Autodesk Fusion 360 part; units mm, degrees
(part 4 of 5)
  spline S150 degree 3 poles (259.5446, 19.7544) (259.234, 19.2928) (259.0786, 18.738) (259.0786, 18.09) knots 0 0 0 0 1 1 1 1
  spline S151 degree 3 poles (259.0786, 18.09) (259.0786, 17.4509) (259.2296, 16.9716) (259.5313, 16.652) knots 0 0 0 0 1 1 1 1
  spline S152 degree 3 poles (259.5313, 16.652) (259.8421, 16.3413) (260.2237, 16.186) (260.6763, 16.186) knots 0 0 0 0 1 1 1 1
  spline S153 degree 3 poles (260.6763, 16.186) (261.3421, 16.186) (261.9812, 16.4168) (262.5937, 16.8784) knots 0 0 0 0 1 1 1 1
  spline S154 degree 3 poles (262.5937, 16.8784) (263.2062, 17.34) (263.7034, 17.9435) (264.0849, 18.6892) knots 0 0 0 0 1 1 1 1
  spline S155 degree 3 poles (264.0849, 18.6892) (264.2803, 18.5028) (264.4577, 18.272) (264.6175, 17.9968) knots 0 0 0 0 1 1 1 1
  spline S156 degree 3 poles (264.6175, 17.9968) (264.3246, 17.3311) (263.8053, 16.6786) (263.0597, 16.0395) knots 0 0 0 0 1 1 1 1
  spline S157 degree 3 poles (263.0597, 16.0395) (262.6869, 15.7289) (262.2431, 15.4759) (261.7282, 15.2806) knots 0 0 0 0 1 1 1 1
  spline S158 degree 3 poles (261.7282, 15.2806) (261.2223, 15.0853) (260.6986, 14.9877) (260.1571, 14.9877) knots 0 0 0 0 1 1 1 1
  spline S159 degree 3 poles (260.1571, 14.9877) (259.2694, 14.9877) (258.5682, 15.2584) (258.0533, 15.7999) knots 0 0 0 0 1 1 1 1
  spline S160 degree 3 poles (258.0533, 15.7999) (257.5031, 16.3857) (257.2278, 17.1358) (257.2278, 18.0501) knots 0 0 0 0 1 1 1 1
  spline S161 degree 3 poles (257.2278, 18.0501) (257.2278, 18.9644) (257.5696, 19.7632) (258.2531, 20.4467) knots 0 0 0 0 1 1 1 1
  spline S162 degree 3 poles (258.2531, 20.4467) (258.9454, 21.1302) (259.7709, 21.472) (260.7296, 21.472) knots 0 0 0 0 1 1 1 1
  spline S163 degree 3 poles (260.7296, 21.472) (261.4132, 21.472) (261.9679, 21.3211) (262.394, 21.0193) knots 0 0 0 0 1 1 1 1
  spline S164 degree 3 poles (262.394, 21.0193) (262.82, 20.7263) (263.0376, 20.3269) (263.0464, 19.8209) knots 0 0 0 0 1 1 1 1
  spline S165 degree 3 poles (263.0464, 19.8209) (263.0464, 19.1374) (262.7713, 18.5827) (262.2209, 18.1566) knots 0 0 0 0 1 1 1 1
  spline S166 degree 3 poles (262.2209, 18.1566) (261.6795, 17.7305) (260.9339, 17.4332) (259.984, 17.2645) knots 0 0 0 0 1 1 1 1
  line L27 (259.984, 17.2645) -> (259.7976, 18.0501)
  spline S167 degree 3 poles (264.5353, 24.8672) (264.7394, 25.0803) (264.988, 25.1868) (265.281, 25.1868) knots 0 0 0 0 1 1 1 1
  spline S168 degree 3 poles (265.281, 25.1868) (265.5739, 25.1868) (265.8223, 25.0803) (266.0266, 24.8672) knots 0 0 0 0 1 1 1 1
  spline S169 degree 3 poles (266.0266, 24.8672) (266.2396, 24.6631) (266.3461, 24.4145) (266.3461, 24.1216) knots 0 0 0 0 1 1 1 1
  spline S170 degree 3 poles (266.3461, 24.1216) (266.3461, 23.8287) (266.2396, 23.5801) (266.0266, 23.376) knots 0 0 0 0 1 1 1 1
  spline S171 degree 3 poles (266.0266, 23.376) (265.8223, 23.1718) (265.5739, 23.0697) (265.281, 23.0697) knots 0 0 0 0 1 1 1 1
  spline S172 degree 3 poles (265.281, 23.0697) (264.988, 23.0697) (264.7394, 23.1718) (264.5353, 23.376) knots 0 0 0 0 1 1 1 1
  spline S173 degree 3 poles (264.5353, 23.376) (264.3311, 23.5801) (264.2291, 23.8287) (264.2291, 24.1216) knots 0 0 0 0 1 1 1 1
  spline S174 degree 3 poles (264.2291, 24.1216) (264.2291, 24.4145) (264.3311, 24.6631) (264.5353, 24.8672) knots 0 0 0 0 1 1 1 1
  spline S175 degree 3 poles (263.9894, 20.966) (264.0781, 21.1258) (264.2468, 21.2456) (264.4954, 21.3255) knots 0 0 0 0 1 1 1 1
  spline S176 degree 3 poles (264.4954, 21.3255) (264.7438, 21.4143) (264.988, 21.4586) (265.2277, 21.4586) knots 0 0 0 0 1 1 1 1
  spline S177 degree 3 poles (265.2277, 21.4586) (265.4761, 21.4586) (265.6937, 21.4276) (265.8801, 21.3654) knots 0 0 0 0 1 1 1 1
  spline S178 degree 3 poles (265.8801, 21.3654) (265.5339, 18.6936) (265.3609, 17.3444) (265.3609, 17.3178) knots 0 0 0 0 1 1 1 1
  spline S179 degree 3 poles (265.3609, 17.3178) (265.3163, 17.1402) (265.2943, 16.9893) (265.2943, 16.8651) knots 0 0 0 0 1 1 1 1
  spline S180 degree 3 poles (265.2943, 16.8651) (265.2943, 16.7497) (265.303, 16.6476) (265.3209, 16.5588) knots 0 0 0 0 1 1 1 1
  spline S181 degree 3 poles (265.3209, 16.5588) (265.3563, 16.328) (265.5161, 16.2126) (265.8002, 16.2126) knots 0 0 0 0 1 1 1 1
  spline S182 degree 3 poles (265.8002, 16.2126) (266.0932, 16.2126) (266.3595, 16.399) (266.5991, 16.7719) knots 0 0 0 0 1 1 1 1
  spline S183 degree 3 poles (266.5991, 16.7719) (266.8475, 17.1535) (267.0339, 17.584) (267.1583, 18.0634) knots 0 0 0 0 1 1 1 1
  spline S184 degree 3 poles (267.1583, 18.0634) (267.2204, 18.0279) (267.3181, 17.9214) (267.4513, 17.7438) knots 0 0 0 0 1 1 1 1
  spline S185 degree 3 poles (267.4513, 17.7438) (267.5844, 17.5663) (267.6643, 17.4332) (267.6909, 17.3444) knots 0 0 0 0 1 1 1 1
  spline S186 degree 3 poles (267.6909, 17.3444) (267.5133, 16.6343) (267.2116, 16.0617) (266.7855, 15.6268) knots 0 0 0 0 1 1 1 1
  spline S187 degree 3 poles (266.7855, 15.6268) (266.3595, 15.1918) (265.8489, 14.9744) (265.2543, 14.9744) knots 0 0 0 0 1 1 1 1
  spline S188 degree 3 poles (265.2543, 14.9744) (264.6596, 14.9744) (264.2158, 15.1208) (263.9229, 15.4137) knots 0 0 0 0 1 1 1 1
  spline S189 degree 3 poles (263.9229, 15.4137) (263.6387, 15.7067) (263.4968, 16.0839) (263.4968, 16.5455) knots 0 0 0 0 1 1 1 1
  spline S190 degree 3 poles (263.4968, 16.5455) (263.4968, 16.6431) (263.5012, 16.7452) (263.5101, 16.8517) knots 0 0 0 0 1 1 1 1
  line L28 (263.5101, 16.8517) -> (263.9894, 20.966)
  line L29 (270.3997, 16.5588) -> (270.7193, 19.528)
  spline S191 degree 3 poles (270.7193, 19.528) (270.7193, 19.7677) (270.6571, 19.9674) (270.5329, 20.1272) knots 0 0 0 0 1 1 1 1
  spline S192 degree 3 poles (270.5329, 20.1272) (270.4085, 20.2869) (270.2, 20.3668) (269.9071, 20.3668) knots 0 0 0 0 1 1 1 1
  spline S193 degree 3 poles (269.9071, 20.3668) (269.6229, 20.3668) (269.3789, 20.2381) (269.1748, 19.9807) knots 0 0 0 0 1 1 1 1
  spline S194 degree 3 poles (269.1748, 19.9807) (268.9794, 19.7322) (268.8552, 19.4171) (268.802, 19.0354) knots 0 0 0 0 1 1 1 1
  spline S195 degree 3 poles (268.802, 19.0354) (268.4824, 16.6032) (268.3137, 15.2806) (268.296, 15.0676) knots 0 0 0 0 1 1 1 1
  line L30 (268.296, 15.0676) -> (266.4985, 15.0676)
  line L31 (266.4985, 15.0676) -> (267.2308, 21.3388)
  spline S196 degree 3 poles (267.2308, 21.3388) (267.6036, 21.4365) (267.8876, 21.4853) (268.083, 21.4853) knots 0 0 0 0 1 1 1 1
  spline S197 degree 3 poles (268.083, 21.4853) (268.6776, 21.4853) (268.9884, 21.2678) (269.015, 20.8328) knots 0 0 0 0 1 1 1 1
  spline S198 degree 3 poles (269.015, 20.8328) (269.4498, 21.2589) (269.9691, 21.472) (270.5728, 21.472) knots 0 0 0 0 1 1 1 1
  spline S199 degree 3 poles (270.5728, 21.472) (271.1853, 21.472) (271.6646, 21.3211) (272.0108, 21.0193) knots 0 0 0 0 1 1 1 1
  spline S200 degree 3 poles (272.0108, 21.0193) (272.357, 20.7175) (272.5301, 20.3358) (272.5301, 19.8742) knots 0 0 0 0 1 1 1 1
  spline S201 degree 3 poles (272.5301, 19.8742) (272.5301, 19.7499) (272.5035, 19.5147) (272.4502, 19.1685) knots 0 0 0 0 1 1 1 1
  spline S202 degree 3 poles (272.4502, 19.1685) (272.2459, 17.8193) (272.144, 17.0337) (272.144, 16.8118) knots 0 0 0 0 1 1 1 1
  spline S203 degree 3 poles (272.144, 16.8118) (272.144, 16.4035) (272.2815, 16.1993) (272.5567, 16.1993) knots 0 0 0 0 1 1 1 1
  spline S204 degree 3 poles (272.5567, 16.1993) (273.1602, 16.1993) (273.6173, 16.8296) (273.9281, 18.09) knots 0 0 0 0 1 1 1 1
  spline S205 degree 3 poles (273.9281, 18.09) (274.2298, 17.7705) (274.4118, 17.5175) (274.474, 17.3311) knots 0 0 0 0 1 1 1 1
  spline S206 degree 3 poles (274.474, 17.3311) (274.0035, 15.7688) (273.1869, 14.9877) (272.0241, 14.9877) knots 0 0 0 0 1 1 1 1
  spline S207 degree 3 poles (272.0241, 14.9877) (271.4737, 14.9877) (271.0655, 15.1563) (270.7992, 15.4936) knots 0 0 0 0 1 1 1 1
  spline S208 degree 3 poles (270.7992, 15.4936) (270.5329, 15.831) (270.3997, 16.186) (270.3997, 16.5588) knots 0 0 0 0 1 1 1 1
  spline S209 degree 3 poles (275.986, 18.0501) (276.5363, 18.1655) (276.9447, 18.3874) (277.211, 18.7158) knots 0 0 0 0 1 1 1 1
  spline S210 degree 3 poles (277.211, 18.7158) (277.486, 19.0442) (277.6237, 19.3594) (277.6237, 19.6611) knots 0 0 0 0 1 1 1 1
  spline S211 degree 3 poles (277.6237, 19.6611) (277.6237, 19.9718) (277.5393, 20.1804) (277.3708, 20.2869) knots 0 0 0 0 1 1 1 1
  spline S212 degree 3 poles (277.3708, 20.2869) (277.211, 20.4023) (277.0333, 20.46) (276.8382, 20.46) knots 0 0 0 0 1 1 1 1
  spline S213 degree 3 poles (276.8382, 20.46) (276.4208, 20.46) (276.0526, 20.2248) (275.733, 19.7544) knots 0 0 0 0 1 1 1 1
  spline S214 degree 3 poles (275.733, 19.7544) (275.4222, 19.2928) (275.267, 18.738) (275.267, 18.09) knots 0 0 0 0 1 1 1 1
  spline S215 degree 3 poles (275.267, 18.09) (275.267, 17.4509) (275.4179, 16.9716) (275.7197, 16.652) knots 0 0 0 0 1 1 1 1
  spline S216 degree 3 poles (275.7197, 16.652) (276.0303, 16.3413) (276.4121, 16.186) (276.8648, 16.186) knots 0 0 0 0 1 1 1 1
  spline S217 degree 3 poles (276.8648, 16.186) (277.5305, 16.186) (278.1696, 16.4168) (278.7821, 16.8784) knots 0 0 0 0 1 1 1 1
  spline S218 degree 3 poles (278.7821, 16.8784) (279.3946, 17.34) (279.8916, 17.9435) (280.2734, 18.6892) knots 0 0 0 0 1 1 1 1
  spline S219 degree 3 poles (280.2734, 18.6892) (280.4685, 18.5028) (280.6462, 18.272) (280.806, 17.9968) knots 0 0 0 0 1 1 1 1
  spline S220 degree 3 poles (280.806, 17.9968) (280.513, 17.3311) (279.9938, 16.6786) (279.2481, 16.0395) knots 0 0 0 0 1 1 1 1
  spline S221 degree 3 poles (279.2481, 16.0395) (278.8753, 15.7289) (278.4314, 15.4759) (277.9167, 15.2806) knots 0 0 0 0 1 1 1 1
  spline S222 degree 3 poles (277.9167, 15.2806) (277.4107, 15.0853) (276.8869, 14.9877) (276.3455, 14.9877) knots 0 0 0 0 1 1 1 1
  spline S223 degree 3 poles (276.3455, 14.9877) (275.4578, 14.9877) (274.7565, 15.2584) (274.2418, 15.7999) knots 0 0 0 0 1 1 1 1
  spline S224 degree 3 poles (274.2418, 15.7999) (273.6913, 16.3857) (273.4163, 17.1358) (273.4163, 18.0501) knots 0 0 0 0 1 1 1 1
  spline S225 degree 3 poles (273.4163, 18.0501) (273.4163, 18.9644) (273.7579, 19.7632) (274.4415, 20.4467) knots 0 0 0 0 1 1 1 1
  spline S226 degree 3 poles (274.4415, 20.4467) (275.1339, 21.1302) (275.9594, 21.472) (276.9181, 21.472) knots 0 0 0 0 1 1 1 1
  spline S227 degree 3 poles (276.9181, 21.472) (277.6015, 21.472) (278.1563, 21.3211) (278.5824, 21.0193) knots 0 0 0 0 1 1 1 1
  spline S228 degree 3 poles (278.5824, 21.0193) (279.0085, 20.7263) (279.2259, 20.3269) (279.2348, 19.8209) knots 0 0 0 0 1 1 1 1
  spline S229 degree 3 poles (279.2348, 19.8209) (279.2348, 19.1374) (278.9596, 18.5827) (278.4093, 18.1566) knots 0 0 0 0 1 1 1 1
  spline S230 degree 3 poles (278.4093, 18.1566) (277.8678, 17.7305) (277.1221, 17.4332) (276.1724, 17.2645) knots 0 0 0 0 1 1 1 1
  line L32 (276.1724, 17.2645) -> (275.986, 18.0501)
  line L33 (231.6876, 10.7897) -> (231.6743, 10.6167)
  spline S231 degree 3 poles (231.6743, 10.6167) (231.337, 8.0247) (231.1151, 6.4269) (231.0085, 5.8233) knots 0 0 0 0 1 1 1 1
  spline S232 degree 3 poles (231.0085, 5.8233) (230.831, 4.8291) (230.7423, 4.0702) (230.7423, 3.5465) knots 0 0 0 0 1 1 1 1
  spline S233 degree 3 poles (230.7423, 3.5465) (230.7423, 3.0316) (230.9642, 2.7743) (231.408, 2.7743) knots 0 0 0 0 1 1 1 1
  spline S234 degree 3 poles (231.408, 2.7743) (231.7808, 2.7743) (232.1137, 3.0406) (232.4066, 3.5731) knots 0 0 0 0 1 1 1 1
  spline S235 degree 3 poles (232.4066, 3.5731) (232.6995, 4.1147) (232.9214, 4.7848) (233.0723, 5.5837) knots 0 0 0 0 1 1 1 1
  spline S236 degree 3 poles (233.0723, 5.5837) (233.383, 7.2525) (233.5383, 8.6949) (233.5383, 9.911) knots 0 0 0 0 1 1 1 1
  spline S237 degree 3 poles (233.5383, 9.911) (233.5383, 10.4791) (233.4895, 10.9717) (233.3919, 11.3889) knots 0 0 0 0 1 1 1 1
  spline S238 degree 3 poles (233.3919, 11.3889) (233.747, 11.6019) (234.173, 11.7085) (234.6701, 11.7085) knots 0 0 0 0 1 1 1 1
  spline S239 degree 3 poles (234.6701, 11.7085) (235.1672, 11.7085) (235.4157, 11.4155) (235.4157, 10.8297) knots 0 0 0 0 1 1 1 1
  spline S240 degree 3 poles (235.4157, 10.8297) (235.4157, 9.9154) (235.2737, 8.5262) (234.9897, 6.6622) knots 0 0 0 0 1 1 1 1
  spline S241 degree 3 poles (234.9897, 6.6622) (234.7589, 5.1087) (234.4393, 3.9682) (234.031, 3.2403) knots 0 0 0 0 1 1 1 1
  spline S242 degree 3 poles (234.031, 3.2403) (233.8446, 2.9297) (233.6316, 2.6322) (233.3919, 2.3482) knots 0 0 0 0 1 1 1 1
  spline S243 degree 3 poles (233.3919, 2.3482) (232.8948, 1.7713) (232.198, 1.4827) (231.3015, 1.4827) knots 0 0 0 0 1 1 1 1
  spline S244 degree 3 poles (231.3015, 1.4827) (230.4138, 1.4827) (229.7792, 1.8645) (229.3975, 2.6278) knots 0 0 0 0 1 1 1 1
  spline S245 degree 3 poles (229.3975, 2.6278) (228.9093, 1.8645) (228.1681, 1.4827) (227.1739, 1.4827) knots 0 0 0 0 1 1 1 1
  spline S246 degree 3 poles (227.1739, 1.4827) (226.5348, 1.4827) (226.0377, 1.6648) (225.6827, 2.0286) knots 0 0 0 0 1 1 1 1
  spline S247 degree 3 poles (225.6827, 2.0286) (225.3365, 2.4014) (225.1634, 2.8941) (225.1634, 3.5066) knots 0 0 0 0 1 1 1 1
  spline S248 degree 3 poles (225.1634, 3.5066) (225.1634, 3.5865) (225.1723, 3.7063) (225.19, 3.8661) knots 0 0 0 0 1 1 1 1
  line L34 (225.19, 3.8661) -> (225.6827, 7.6208)
  spline S249 degree 3 poles (225.6827, 7.6208) (224.7329, 8.3043) (224.258, 9.0721) (224.258, 9.9243) knots 0 0 0 0 1 1 1 1
  spline S250 degree 3 poles (224.258, 9.9243) (224.258, 10.4658) (224.4444, 10.8963) (224.8172, 11.2158) knots 0 0 0 0 1 1 1 1
  spline S251 degree 3 poles (224.8172, 11.2158) (225.19, 11.5354) (225.6427, 11.6952) (226.1753, 11.6952) knots 0 0 0 0 1 1 1 1
  spline S252 degree 3 poles (226.1753, 11.6952) (227.3381, 11.6952) (227.9195, 11.1182) (227.9195, 9.9642) knots 0 0 0 0 1 1 1 1
  spline S253 degree 3 poles (227.9195, 9.9642) (227.9195, 9.9465) (227.9151, 9.9243) (227.9062, 9.8977) knots 0 0 0 0 1 1 1 1
  spline S254 degree 3 poles (227.9062, 9.8977) (227.9062, 9.871) (227.9018, 9.8267) (227.8929, 9.7645) knots 0 0 0 0 1 1 1 1
  spline S255 degree 3 poles (227.8929, 9.7645) (227.8929, 9.7113) (227.884, 9.6447) (227.8663, 9.5648) knots 0 0 0 0 1 1 1 1
  spline S256 degree 3 poles (227.8663, 9.5648) (227.8574, 9.4938) (227.8396, 9.3828) (227.813, 9.2319) knots 0 0 0 0 1 1 1 1
  spline S257 degree 3 poles (227.813, 9.2319) (227.7953, 9.081) (227.7731, 8.9124) (227.7464, 8.726) knots 0 0 0 0 1 1 1 1
  spline S258 degree 3 poles (227.7464, 8.726) (227.7198, 8.5484) (227.6843, 8.3088) (227.6399, 8.007) knots 0 0 0 0 1 1 1 1
  spline S259 degree 3 poles (227.6399, 8.007) (227.5955, 7.7052) (227.5467, 7.3767) (227.4935, 7.0217) knots 0 0 0 0 1 1 1 1
  spline S260 degree 3 poles (227.4935, 7.0217) (227.4491, 6.6755) (227.3914, 6.2494) (227.3204, 5.7434) knots 0 0 0 0 1 1 1 1
  spline S261 degree 3 poles (227.3204, 5.7434) (227.2494, 5.2375) (227.1872, 4.807) (227.134, 4.4519) knots 0 0 0 0 1 1 1 1
  spline S262 degree 3 poles (227.134, 4.4519) (227.0807, 4.0968) (227.0541, 3.8394) (227.0541, 3.6797) knots 0 0 0 0 1 1 1 1
  spline S263 degree 3 poles (227.0541, 3.6797) (227.0541, 3.0849) (227.2849, 2.7876) (227.7464, 2.7876) knots 0 0 0 0 1 1 1 1
  spline S264 degree 3 poles (227.7464, 2.7876) (228.3855, 2.7876) (228.7806, 3.369) (228.9314, 4.5318) knots 0 0 0 0 1 1 1 1
  line L35 (228.9314, 4.5318) -> (229.7836, 11.2558)
  spline S265 degree 3 poles (229.7836, 11.2558) (230.0765, 11.3889) (230.4271, 11.4555) (230.8355, 11.4555) knots 0 0 0 0 1 1 1 1
  spline S266 degree 3 poles (230.8355, 11.4555) (231.4036, 11.4555) (231.6876, 11.2336) (231.6876, 10.7897) knots 0 0 0 0 1 1 1 1
  spline S267 degree 3 poles (225.656, 10.63) (225.4874, 10.63) (225.3631, 10.5678) (225.2832, 10.4436) knots 0 0 0 0 1 1 1 1
  spline S268 degree 3 poles (225.2832, 10.4436) (225.2033, 10.3193) (225.1634, 10.1773) (225.1634, 10.0175) knots 0 0 0 0 1 1 1 1
  spline S269 degree 3 poles (225.1634, 10.0175) (225.1634, 9.6181) (225.3853, 9.2053) (225.8291, 8.7792) knots 0 0 0 0 1 1 1 1
  line L36 (225.8291, 8.7792) -> (225.8957, 9.3118)
  spline S270 degree 3 poles (225.8957, 9.3118) (225.9312, 9.6047) (225.9489, 9.8977) (225.9489, 10.1906) knots 0 0 0 0 1 1 1 1
  spline S271 degree 3 poles (225.9489, 10.1906) (225.9578, 10.4835) (225.8602, 10.63) (225.656, 10.63) knots 0 0 0 0 1 1 1 1
  spline S272 degree 3 poles (238.1872, 4.5451) (238.7375, 4.6606) (239.1458, 4.8824) (239.4121, 5.2109) knots 0 0 0 0 1 1 1 1
  spline S273 degree 3 poles (239.4121, 5.2109) (239.6874, 5.5393) (239.8249, 5.8543) (239.8249, 6.1562) knots 0 0 0 0 1 1 1 1
  spline S274 degree 3 poles (239.8249, 6.1562) (239.8249, 6.4669) (239.7406, 6.6755) (239.5719, 6.782) knots 0 0 0 0 1 1 1 1
  spline S275 degree 3 poles (239.5719, 6.782) (239.4121, 6.8974) (239.2347, 6.9551) (239.0393, 6.9551) knots 0 0 0 0 1 1 1 1
  spline S276 degree 3 poles (239.0393, 6.9551) (238.6221, 6.9551) (238.2537, 6.7199) (237.9342, 6.2494) knots 0 0 0 0 1 1 1 1
  spline S277 degree 3 poles (237.9342, 6.2494) (237.6235, 5.7878) (237.4682, 5.2331) (237.4682, 4.5851) knots 0 0 0 0 1 1 1 1
  spline S278 degree 3 poles (237.4682, 4.5851) (237.4682, 3.946) (237.6191, 3.4666) (237.9209, 3.1471) knots 0 0 0 0 1 1 1 1
  spline S279 degree 3 poles (237.9209, 3.1471) (238.2315, 2.8365) (238.6132, 2.6811) (239.066, 2.6811) knots 0 0 0 0 1 1 1 1
  spline S280 degree 3 poles (239.066, 2.6811) (239.7317, 2.6811) (240.3708, 2.9118) (240.9833, 3.3734) knots 0 0 0 0 1 1 1 1
  spline S281 degree 3 poles (240.9833, 3.3734) (241.5958, 3.8351) (242.0928, 4.4386) (242.4745, 5.1842) knots 0 0 0 0 1 1 1 1
  spline S282 degree 3 poles (242.4745, 5.1842) (242.6699, 4.9978) (242.8473, 4.7671) (243.0071, 4.4919) knots 0 0 0 0 1 1 1 1
  spline S283 degree 3 poles (243.0071, 4.4919) (242.7142, 3.8261) (242.1949, 3.1737) (241.4493, 2.5346) knots 0 0 0 0 1 1 1 1
  spline S284 degree 3 poles (241.4493, 2.5346) (241.0765, 2.224) (240.6327, 1.971) (240.1178, 1.7757) knots 0 0 0 0 1 1 1 1
  spline S285 degree 3 poles (240.1178, 1.7757) (239.6119, 1.5803) (239.0882, 1.4827) (238.5467, 1.4827) knots 0 0 0 0 1 1 1 1
  spline S286 degree 3 poles (238.5467, 1.4827) (237.659, 1.4827) (236.9578, 1.7534) (236.4429, 2.2949) knots 0 0 0 0 1 1 1 1
  spline S287 degree 3 poles (236.4429, 2.2949) (235.8926, 2.8808) (235.6174, 3.6308) (235.6174, 4.5451) knots 0 0 0 0 1 1 1 1
  spline S288 degree 3 poles (235.6174, 4.5451) (235.6174, 5.4595) (235.9592, 6.2583) (236.6427, 6.9418) knots 0 0 0 0 1 1 1 1
  spline S289 degree 3 poles (236.6427, 6.9418) (237.335, 7.6253) (238.1605, 7.967) (239.1192, 7.967) knots 0 0 0 0 1 1 1 1
  spline S290 degree 3 poles (239.1192, 7.967) (239.8026, 7.967) (240.3575, 7.8161) (240.7836, 7.5143) knots 0 0 0 0 1 1 1 1
  spline S291 degree 3 poles (240.7836, 7.5143) (241.2096, 7.2214) (241.427, 6.822) (241.436, 6.316) knots 0 0 0 0 1 1 1 1
  spline S292 degree 3 poles (241.436, 6.316) (241.436, 5.6326) (241.1607, 5.0777) (240.6105, 4.6516) knots 0 0 0 0 1 1 1 1
  spline S293 degree 3 poles (240.6105, 4.6516) (240.0689, 4.2256) (239.3233, 3.9283) (238.3736, 3.7595) knots 0 0 0 0 1 1 1 1
  line L37 (238.3736, 3.7595) -> (238.1872, 4.5451)
  spline S294 degree 3 poles (245.8407, 6.2228) (245.8407, 6.6134) (245.6588, 6.8086) (245.2948, 6.8086) knots 0 0 0 0 1 1 1 1
  spline S295 degree 3 poles (245.2948, 6.8086) (244.9399, 6.8086) (244.6557, 6.5779) (244.4426, 6.1163) knots 0 0 0 0 1 1 1 1
  spline S296 degree 3 poles (244.4426, 6.1163) (245.4013, 5.3617) (245.8806, 4.5141) (245.8806, 3.5731) knots 0 0 0 0 1 1 1 1
  spline S297 degree 3 poles (245.8806, 3.5731) (245.8806, 2.8897) (245.6899, 2.3704) (245.3081, 2.0153) knots 0 0 0 0 1 1 1 1
  spline S298 degree 3 poles (245.3081, 2.0153) (244.9265, 1.6602) (244.4472, 1.4827) (243.8701, 1.4827) knots 0 0 0 0 1 1 1 1
  spline S299 degree 3 poles (243.8701, 1.4827) (243.2932, 1.4827) (242.8715, 1.6602) (242.6052, 2.0153) knots 0 0 0 0 1 1 1 1
  spline S300 degree 3 poles (242.6052, 2.0153) (242.3389, 2.3792) (242.2058, 2.8365) (242.2058, 3.3867) knots 0 0 0 0 1 1 1 1
  spline S301 degree 3 poles (242.2058, 3.3867) (242.2058, 3.5555) (242.2103, 3.6797) (242.2191, 3.7595) knots 0 0 0 0 1 1 1 1
  line L38 (242.2191, 3.7595) -> (242.6851, 7.8206)
  spline S302 degree 3 poles (242.6851, 7.8206) (243.0047, 7.9182) (243.3288, 7.967) (243.6571, 7.967) knots 0 0 0 0 1 1 1 1
  spline S303 degree 3 poles (243.6571, 7.967) (244.1986, 7.967) (244.4693, 7.7673) (244.4693, 7.3679) knots 0 0 0 0 1 1 1 1
  line L39 (244.4693, 7.3679) -> (244.4693, 7.3412)
  spline S304 degree 3 poles (244.4693, 7.3412) (244.8244, 7.7584) (245.2771, 7.967) (245.8274, 7.967) knots 0 0 0 0 1 1 1 1
  spline S305 degree 3 poles (245.8274, 7.967) (246.2268, 7.967) (246.5376, 7.8738) (246.7594, 7.6874) knots 0 0 0 0 1 1 1 1
  spline S306 degree 3 poles (246.7594, 7.6874) (246.9814, 7.5099) (247.0923, 7.2702) (247.0923, 6.9684) knots 0 0 0 0 1 1 1 1
  spline S307 degree 3 poles (247.0923, 6.9684) (247.0923, 6.6666) (246.977, 6.4181) (246.7461, 6.2228) knots 0 0 0 0 1 1 1 1
  spline S308 degree 3 poles (246.7461, 6.2228) (246.5243, 6.0364) (246.2314, 5.9432) (245.8673, 5.9432) knots 0 0 0 0 1 1 1 1
  spline S309 degree 3 poles (245.8673, 5.9432) (245.8496, 5.9432) (245.8319, 5.9432) (245.8141, 5.9432) knots 0 0 0 0 1 1 1 1
  spline S310 degree 3 poles (245.8141, 5.9432) (245.8319, 6.0407) (245.8407, 6.1339) (245.8407, 6.2228) knots 0 0 0 0 1 1 1 1
  spline S311 degree 3 poles (245.0152, 3.6397) (245.0152, 4.1546) (244.7489, 4.6693) (244.2163, 5.1842) knots 0 0 0 0 1 1 1 1
  spline S312 degree 3 poles (244.2163, 5.1842) (244.0565, 3.906) (243.9766, 3.2625) (243.9766, 3.2536) knots 0 0 0 0 1 1 1 1
  spline S313 degree 3 poles (243.9766, 3.2536) (243.9766, 2.8808) (244.1277, 2.6944) (244.4293, 2.6944) knots 0 0 0 0 1 1 1 1
  spline S314 degree 3 poles (244.4293, 2.6944) (244.82, 2.6944) (245.0152, 3.0095) (245.0152, 3.6397) knots 0 0 0 0 1 1 1 1
  spline S315 degree 3 poles (251.3013, 7.9803) (251.9404, 7.9803) (252.4906, 7.7185) (252.9523, 7.1948) knots 0 0 0 0 1 1 1 1
  spline S316 degree 3 poles (252.9523, 7.1948) (253.4139, 6.6711) (253.6446, 6.0586) (253.6446, 5.3573) knots 0 0 0 0 1 1 1 1
  spline S317 degree 3 poles (253.6446, 5.3573) (253.6446, 5.2597) (253.6403, 5.1576) (253.6313, 5.0511) knots 0 0 0 0 1 1 1 1
  spline S318 degree 3 poles (253.6313, 5.0511) (253.5338, 3.8883) (253.1431, 3.0006) (252.4596, 2.3881) knots 0 0 0 0 1 1 1 1
  spline S319 degree 3 poles (252.4596, 2.3881) (251.7762, 1.7846) (250.8841, 1.4827) (249.7834, 1.4827) knots 0 0 0 0 1 1 1 1
  spline S320 degree 3 poles (249.7834, 1.4827) (249.3396, 1.5004) (248.9535, 1.5803) (248.625, 1.7224) knots 0 0 0 0 1 1 1 1
  spline S321 degree 3 poles (248.625, 1.7224) (248.2965, 1.8645) (248.0525, 2.0419) (247.8927, 2.255) knots 0 0 0 0 1 1 1 1
  spline S322 degree 3 poles (247.8927, 2.255) (247.5908, 2.6455) (247.44, 2.9917) (247.44, 3.2935) knots 0 0 0 0 1 1 1 1
  spline S323 degree 3 poles (247.44, 3.2935) (247.44, 3.6041) (247.4843, 4.1014) (247.5731, 4.7848) knots 0 0 0 0 1 1 1 1
  spline S324 degree 3 poles (247.5731, 4.7848) (247.7595, 6.1872) (248.0258, 8.4552) (248.372, 11.5886) knots 0 0 0 0 1 1 1 1
  spline S325 degree 3 poles (248.372, 11.5886) (248.5584, 11.6596) (248.807, 11.6952) (249.1176, 11.6952) knots 0 0 0 0 1 1 1 1
  spline S326 degree 3 poles (249.1176, 11.6952) (249.8277, 11.6952) (250.1828, 11.491) (250.1828, 11.0827) knots 0 0 0 0 1 1 1 1
  line L40 (250.1828, 11.0827) -> (249.7301, 7.541)
  spline S327 degree 3 poles (249.7301, 7.541) (250.1472, 7.8339) (250.6711, 7.9803) (251.3013, 7.9803) knots 0 0 0 0 1 1 1 1
  spline S328 degree 3 poles (249.2375, 3.3867) (249.2375, 3.1826) (249.313, 3.0095) (249.4638, 2.8675) knots 0 0 0 0 1 1 1 1
  spline S329 degree 3 poles (249.4638, 2.8675) (249.6236, 2.7343) (249.841, 2.6677) (250.1162, 2.6677) knots 0 0 0 0 1 1 1 1
  spline S330 degree 3 poles (250.1162, 2.6677) (250.5689, 2.6677) (250.9418, 2.8764) (251.2347, 3.2935) knots 0 0 0 0 1 1 1 1
  spline S331 degree 3 poles (251.2347, 3.2935) (251.5898, 3.7995) (251.7673, 4.4563) (251.7673, 5.2641) knots 0 0 0 0 1 1 1 1
  spline S332 degree 3 poles (251.7673, 5.2641) (251.7673, 5.6546) (251.6784, 6.0008) (251.501, 6.3027) knots 0 0 0 0 1 1 1 1
  spline S333 degree 3 poles (251.501, 6.3027) (251.3235, 6.6045) (251.0483, 6.7554) (250.6755, 6.7554) knots 0 0 0 0 1 1 1 1
  spline S334 degree 3 poles (250.6755, 6.7554) (250.1695, 6.7554) (249.7834, 6.4536) (249.5171, 5.85) knots 0 0 0 0 1 1 1 1
  line L41 (249.5171, 5.85) -> (249.4106, 5.0511)
  spline S335 degree 3 poles (249.4106, 5.0511) (249.2951, 4.1546) (249.2375, 3.5998) (249.2375, 3.3867) knots 0 0 0 0 1 1 1 1
  spline S336 degree 3 poles (260.1517, 7.8339) (259.7879, 4.9579) (259.6058, 3.4267) (259.6058, 3.2403) knots 0 0 0 0 1 1 1 1
  spline S337 degree 3 poles (259.6058, 3.2403) (259.6058, 2.8852) (259.7346, 2.7077) (259.992, 2.7077) knots 0 0 0 0 1 1 1 1
  spline S338 degree 3 poles (259.992, 2.7077) (260.2229, 2.7077) (260.4713, 2.8631) (260.7376, 3.1737) knots 0 0 0 0 1 1 1 1
  spline S339 degree 3 poles (260.7376, 3.1737) (261.0128, 3.4933) (261.2302, 3.9682) (261.39, 4.5984) knots 0 0 0 0 1 1 1 1
  spline S340 degree 3 poles (261.39, 4.5984) (261.6829, 4.2788) (261.8606, 4.0302) (261.9226, 3.8528) knots 0 0 0 0 1 1 1 1
  spline S341 degree 3 poles (261.9226, 3.8528) (261.7185, 2.9917) (261.3946, 2.3838) (260.9506, 2.0286) knots 0 0 0 0 1 1 1 1
  spline S342 degree 3 poles (260.9506, 2.0286) (260.5069, 1.6735) (260.0498, 1.496) (259.5792, 1.496) knots 0 0 0 0 1 1 1 1
  spline S343 degree 3 poles (259.5792, 1.496) (258.807, 1.496) (258.2877, 1.7933) (258.0214, 2.3881) knots 0 0 0 0 1 1 1 1
  spline S344 degree 3 poles (258.0214, 2.3881) (257.5599, 1.7933) (256.9429, 1.496) (256.1706, 1.496) knots 0 0 0 0 1 1 1 1
  spline S345 degree 3 poles (256.1706, 1.496) (255.5315, 1.496) (255.0389, 1.6558) (254.6927, 1.9754) knots 0 0 0 0 1 1 1 1
  spline S346 degree 3 poles (254.6927, 1.9754) (254.3465, 2.2949) (254.1734, 2.7121) (254.1734, 3.227) knots 0 0 0 0 1 1 1 1
  spline S347 degree 3 poles (254.1734, 3.227) (254.1734, 3.3512) (254.1957, 3.5688) (254.24, 3.8794) knots 0 0 0 0 1 1 1 1
  spline S348 degree 3 poles (254.24, 3.8794) (254.4443, 5.5304) (254.5995, 6.8442) (254.706, 7.8206) knots 0 0 0 0 1 1 1 1
  spline S349 degree 3 poles (254.706, 7.8206) (254.9813, 7.9182) (255.2342, 7.967) (255.465, 7.967) knots 0 0 0 0 1 1 1 1
  spline S350 degree 3 poles (255.465, 7.967) (255.6959, 7.967) (255.869, 7.9581) (255.9842, 7.9404) knots 0 0 0 0 1 1 1 1
  spline S351 degree 3 poles (255.9842, 7.9404) (256.0997, 7.9226) (256.2106, 7.8561) (256.3171, 7.7407) knots 0 0 0 0 1 1 1 1
  spline S352 degree 3 poles (256.3171, 7.7407) (256.4236, 7.6253) (256.4769, 7.4611) (256.4769, 7.248) knots 0 0 0 0 1 1 1 1
  line L42 (256.4769, 7.248) -> (256.0375, 3.8528)
  spline S353 degree 3 poles (256.0375, 3.8528) (256.0198, 3.7462) (256.0109, 3.6487) (256.0109, 3.5598) knots 0 0 0 0 1 1 1 1
  spline S354 degree 3 poles (256.0109, 3.5598) (256.0109, 3.0362) (256.2505, 2.7743) (256.7299, 2.7743) knots 0 0 0 0 1 1 1 1
  spline S355 degree 3 poles (256.7299, 2.7743) (257.1738, 2.7743) (257.5421, 2.9917) (257.835, 3.4267) knots 0 0 0 0 1 1 1 1
  spline S356 degree 3 poles (257.835, 3.4267) (257.835, 3.5243) (257.8439, 3.6797) (257.8616, 3.8927) knots 0 0 0 0 1 1 1 1
  line L43 (257.8616, 3.8927) -> (258.301, 7.4344)
  spline S357 degree 3 poles (258.301, 7.4344) (258.3632, 7.5853) (258.4963, 7.7096) (258.7004, 7.8072) knots 0 0 0 0 1 1 1 1
  spline S358 degree 3 poles (258.7004, 7.8072) (258.9047, 7.9138) (259.1577, 7.967) (259.4594, 7.967) knots 0 0 0 0 1 1 1 1
  spline S359 degree 3 poles (259.4594, 7.967) (259.7702, 7.967) (260.0009, 7.9226) (260.1517, 7.8339) knots 0 0 0 0 1 1 1 1
  line L44 (264.7566, 3.0539) -> (265.0761, 6.0231)
  spline S360 degree 3 poles (265.0761, 6.0231) (265.0761, 6.2627) (265.0139, 6.4625) (264.8897, 6.6222) knots 0 0 0 0 1 1 1 1
  spline S361 degree 3 poles (264.8897, 6.6222) (264.7653, 6.782) (264.5568, 6.8619) (264.2639, 6.8619) knots 0 0 0 0 1 1 1 1
  spline S362 degree 3 poles (264.2639, 6.8619) (263.9797, 6.8619) (263.7357, 6.7332) (263.5316, 6.4758) knots 0 0 0 0 1 1 1 1
  spline S363 degree 3 poles (263.5316, 6.4758) (263.3363, 6.2271) (263.212, 5.9122) (263.1588, 5.5304) knots 0 0 0 0 1 1 1 1
  spline S364 degree 3 poles (263.1588, 5.5304) (262.8392, 3.0982) (262.6705, 1.7757) (262.6528, 1.5626) knots 0 0 0 0 1 1 1 1
  line L45 (262.6528, 1.5626) -> (260.8553, 1.5626)
  line L46 (260.8553, 1.5626) -> (261.5876, 7.8339)
  spline S365 degree 3 poles (261.5876, 7.8339) (261.9605, 7.9315) (262.2444, 7.9803) (262.4398, 7.9803) knots 0 0 0 0 1 1 1 1
  spline S366 degree 3 poles (262.4398, 7.9803) (263.0344, 7.9803) (263.3452, 7.7629) (263.3718, 7.3279) knots 0 0 0 0 1 1 1 1
  spline S367 degree 3 poles (263.3718, 7.3279) (263.8066, 7.754) (264.3259, 7.967) (264.9296, 7.967) knots 0 0 0 0 1 1 1 1
  spline S368 degree 3 poles (264.9296, 7.967) (265.5421, 7.967) (266.0215, 7.8161) (266.3676, 7.5143) knots 0 0 0 0 1 1 1 1
  spline S369 degree 3 poles (266.3676, 7.5143) (266.7138, 7.2125) (266.8869, 6.8308) (266.8869, 6.3693) knots 0 0 0 0 1 1 1 1
  spline S370 degree 3 poles (266.8869, 6.3693) (266.8869, 6.245) (266.8603, 6.0097) (266.807, 5.6636) knots 0 0 0 0 1 1 1 1
  spline S371 degree 3 poles (266.807, 5.6636) (266.6027, 4.3144) (266.5008, 3.5288) (266.5008, 3.3068) knots 0 0 0 0 1 1 1 1
  spline S372 degree 3 poles (266.5008, 3.3068) (266.5008, 2.8985) (266.6383, 2.6944) (266.9135, 2.6944) knots 0 0 0 0 1 1 1 1
  spline S373 degree 3 poles (266.9135, 2.6944) (267.5171, 2.6944) (267.9742, 3.3245) (268.285, 4.5851) knots 0 0 0 0 1 1 1 1
  spline S374 degree 3 poles (268.285, 4.5851) (268.5866, 4.2655) (268.7687, 4.0125) (268.8309, 3.8261) knots 0 0 0 0 1 1 1 1
  spline S375 degree 3 poles (268.8309, 3.8261) (268.3603, 2.2639) (267.5437, 1.4827) (266.381, 1.4827) knots 0 0 0 0 1 1 1 1
  spline S376 degree 3 poles (266.381, 1.4827) (265.8305, 1.4827) (265.4223, 1.6514) (265.156, 1.9887) knots 0 0 0 0 1 1 1 1
  spline S377 degree 3 poles (265.156, 1.9887) (264.8897, 2.3259) (264.7566, 2.6811) (264.7566, 3.0539) knots 0 0 0 0 1 1 1 1
  spline S378 degree 3 poles (271.448, 7.967) (271.9361, 7.967) (272.3844, 7.8871) (272.7928, 7.7274) knots 0 0 0 0 1 1 1 1
  spline S379 degree 3 poles (272.7928, 7.7274) (273.0678, 7.896) (273.3564, 7.9803) (273.6582, 7.9803) knots 0 0 0 0 1 1 1 1
  spline S380 degree 3 poles (273.6582, 7.9803) (273.9599, 7.9803) (274.1996, 7.9404) (274.3772, 7.8605) knots 0 0 0 0 1 1 1 1
  line L47 (274.3772, 7.8605) -> (273.8979, 4.1057)
  spline S381 degree 3 poles (273.8979, 4.1057) (274.5547, 4.6117) (275.0517, 5.0733) (275.3891, 5.4905) knots 0 0 0 0 1 1 1 1
  line L48 (275.3891, 5.4905) -> (275.7753, 4.6783)
  spline S382 degree 3 poles (275.7753, 4.6783) (275.2693, 4.1457) (274.5946, 3.5775) (273.7514, 2.974) knots 0 0 0 0 1 1 1 1
  line L49 (273.7514, 2.974) -> (273.3919, 0.1912)
  spline S383 degree 3 poles (273.3919, 0.1912) (273.2942, -0.6433) (273.0191, -1.2824) (272.5664, -1.7261) knots 0 0 0 0 1 1 1 1
  spline S384 degree 3 poles (272.5664, -1.7261) (272.1225, -2.1788) (271.5456, -2.4052) (270.8355, -2.4052) knots 0 0 0 0 1 1 1 1
  spline S385 degree 3 poles (270.8355, -2.4052) (270.4271, -2.4052) (270.0277, -2.272) (269.6372, -2.0057) knots 0 0 0 0 1 1 1 1
  spline S386 degree 3 poles (269.6372, -2.0057) (269.2288, -1.7217) (269.0247, -1.2645) (269.0247, -0.6343) knots 0 0 0 0 1 1 1 1
  spline S387 degree 3 poles (269.0247, -0.6343) (269.0247, 0.1379) (269.3929, 0.8436) (270.1298, 1.4827) knots 0 0 0 0 1 1 1 1
  spline S388 degree 3 poles (270.1298, 1.4827) (269.4995, 1.527) (268.9581, 1.789) (268.5054, 2.2683) knots 0 0 0 0 1 1 1 1
  spline S389 degree 3 poles (268.5054, 2.2683) (268.0527, 2.7476) (267.8264, 3.3734) (267.8264, 4.1457) knots 0 0 0 0 1 1 1 1
  spline S390 degree 3 poles (267.8264, 4.1457) (267.8264, 5.3084) (268.168, 6.2361) (268.8516, 6.9285) knots 0 0 0 0 1 1 1 1
  spline S391 degree 3 poles (268.8516, 6.9285) (269.535, 7.6208) (270.4005, 7.967) (271.448, 7.967) knots 0 0 0 0 1 1 1 1
  spline S392 degree 3 poles (271.6477, 6.9285) (271.0795, 6.9285) (270.6268, 6.711) (270.2896, 6.276) knots 0 0 0 0 1 1 1 1
  spline S393 degree 3 poles (270.2896, 6.276) (269.9611, 5.85) (269.7657, 5.2109) (269.7037, 4.3587) knots 0 0 0 0 1 1 1 1
  spline S394 degree 3 poles (269.7037, 4.3587) (269.6948, 4.2788) (269.6904, 4.2033) (269.6904, 4.1324) knots 0 0 0 0 1 1 1 1
  spline S395 degree 3 poles (269.6904, 4.1324) (269.6904, 3.6973) (269.7924, 3.3512) (269.9967, 3.0938) knots 0 0 0 0 1 1 1 1
  spline S396 degree 3 poles (269.9967, 3.0938) (270.2097, 2.8365) (270.4804, 2.7077) (270.8089, 2.7077) knots 0 0 0 0 1 1 1 1
  spline S397 degree 3 poles (270.8089, 2.7077) (271.3681, 2.7077) (271.7896, 3.0982) (272.0738, 3.8794) knots 0 0 0 0 1 1 1 1
  line L50 (272.0738, 3.8794) -> (272.4066, 6.7687)
  spline S398 degree 3 poles (272.4066, 6.7687) (272.1314, 6.8752) (271.8784, 6.9285) (271.6477, 6.9285) knots 0 0 0 0 1 1 1 1
  spline S399 degree 3 poles (270.0499, -0.4346) (270.0499, -0.6743) (270.1165, -0.8607) (270.2496, -0.9938) knots 0 0 0 0 1 1 1 1
  spline S400 degree 3 poles (270.2496, -0.9938) (270.3915, -1.1359) (270.5513, -1.2068) (270.729, -1.2068) knots 0 0 0 0 1 1 1 1
  spline S401 degree 3 poles (270.729, -1.2068) (271.226, -1.2068) (271.5145, -0.8917) (271.5944, -0.2615) knots 0 0 0 0 1 1 1 1
  line L51 (271.5944, -0.2615) -> (271.8208, 1.7357)
  spline S402 degree 3 poles (271.8208, 1.7357) (270.6402, 1.0344) (270.0499, 0.311) (270.0499, -0.4346) knots 0 0 0 0 1 1 1 1
  spline S403 degree 3 poles (230.1003, 16.5932) (229.6981, 16.9277) (229.2899, 16.9441) (228.9476, 16.8238) knots 0 0 0 0 1 1 1 1
  spline S404 degree 3 poles (228.9476, 16.8238) (228.7165, 16.7425) (228.517, 16.5999) (228.3674, 16.4563) knots 0 0 0 0 1 1 1 1
  line L52 (228.3674, 16.4563) -> (228.3674, 17.472)
  spline S405 degree 3 poles (228.3674, 17.472) (228.4813, 17.44) (228.6086, 17.4278) (228.7401, 17.4288) knots 0 0 0 0 1 1 1 1
  spline S406 degree 3 poles (228.7401, 17.4288) (228.9289, 17.4302) (229.1344, 17.4585) (229.3365, 17.5008) knots 0 0 0 0 1 1 1 1
  spline S407 degree 3 poles (229.3365, 17.5008) (229.6898, 17.5747) (230.0407, 17.6927) (230.2884, 17.7918) knots 0 0 0 0 1 1 1 1
  spline S408 degree 3 poles (230.2884, 17.7918) (230.3819, 17.4435) (230.468, 17.0095) (230.459, 16.7175) knots 0 0 0 0 1 1 1 1
  spline S409 degree 3 poles (230.459, 16.7175) (230.4566, 16.638) (230.4471, 16.5744) (230.4317, 16.5283) knots 0 0 0 0 1 1 1 1
  spline S410 degree 3 poles (230.4317, 16.5283) (230.4161, 16.4815) (230.3982, 16.4636) (230.3866, 16.457) knots 0 0 0 0 1 1 1 1
  spline S411 degree 3 poles (230.3866, 16.457) (230.3774, 16.4519) (230.3561, 16.4447) (230.3077, 16.4615) knots 0 0 0 0 1 1 1 1
  spline S412 degree 3 poles (230.3077, 16.4615) (230.258, 16.4789) (230.1898, 16.5188) (230.1003, 16.5932) knots 0 0 0 0 1 1 1 1
  spline S413 degree 3 poles (235.9582, 4.295) (235.7441, 4.4959) (235.5256, 4.6047) (235.3108, 4.6431) knots 0 0 0 0 1 1 1 1
  spline S414 degree 3 poles (235.3108, 4.6431) (235.0964, 4.6815) (234.8926, 4.6482) (234.7093, 4.5756) knots 0 0 0 0 1 1 1 1
  spline S415 degree 3 poles (234.7093, 4.5756) (234.4543, 4.4744) (234.2356, 4.2958) (234.0737, 4.1181) knots 0 0 0 0 1 1 1 1
  line L53 (234.0737, 4.1181) -> (234.0737, 5.4125)
  spline S416 degree 3 poles (234.0737, 5.4125) (234.1989, 5.3716) (234.3398, 5.3562) (234.4854, 5.3573) knots 0 0 0 0 1 1 1 1
  spline S417 degree 3 poles (234.4854, 5.3573) (234.6904, 5.359) (234.9132, 5.3938) (235.1323, 5.4454) knots 0 0 0 0 1 1 1 1
  spline S418 degree 3 poles (235.1323, 5.4454) (235.5164, 5.5361) (235.8979, 5.6811) (236.1663, 5.8024) knots 0 0 0 0 1 1 1 1
  spline S419 degree 3 poles (236.1663, 5.8024) (236.2691, 5.3735) (236.3655, 4.8316) (236.3555, 4.466) knots 0 0 0 0 1 1 1 1
  spline S420 degree 3 poles (236.3555, 4.466) (236.3528, 4.3671) (236.3424, 4.2861) (236.3246, 4.2258) knots 0 0 0 0 1 1 1 1
  spline S421 degree 3 poles (236.3246, 4.2258) (236.3062, 4.1637) (236.284, 4.1373) (236.2686, 4.1274) knots 0 0 0 0 1 1 1 1
  spline S422 degree 3 poles (236.2686, 4.1274) (236.2584, 4.1209) (236.2364, 4.1124) (236.1845, 4.1327) knots 0 0 0 0 1 1 1 1
  spline S423 degree 3 poles (236.1845, 4.1327) (236.1304, 4.154) (236.0558, 4.2033) (235.9582, 4.295) knots 0 0 0 0 1 1 1 1
  spline S424 degree 3 poles (247.561, 2.9635) (247.347, 3.1644) (247.1284, 3.2732) (246.9137, 3.3116) knots 0 0 0 0 1 1 1 1
  spline S425 degree 3 poles (246.9137, 3.3116) (246.6993, 3.35) (246.4954, 3.3167) (246.3122, 3.2441) knots 0 0 0 0 1 1 1 1
  spline S426 degree 3 poles (246.3122, 3.2441) (246.0572, 3.1429) (245.8384, 2.9643) (245.6765, 2.7866) knots 0 0 0 0 1 1 1 1
  line L54 (245.6765, 2.7866) -> (245.6765, 4.081)
  spline S427 degree 3 poles (245.6765, 4.081) (245.8019, 4.0401) (245.9426, 4.0247) (246.0883, 4.0258) knots 0 0 0 0 1 1 1 1
  spline S428 degree 3 poles (246.0883, 4.0258) (246.2932, 4.0276) (246.5161, 4.0624) (246.7351, 4.1139) knots 0 0 0 0 1 1 1 1
  spline S429 degree 3 poles (246.7351, 4.1139) (247.1193, 4.2046) (247.5007, 4.3496) (247.7692, 4.4709) knots 0 0 0 0 1 1 1 1
  spline S430 degree 3 poles (247.7692, 4.4709) (247.8719, 4.042) (247.9684, 3.5001) (247.9583, 3.1345) knots 0 0 0 0 1 1 1 1
  spline S431 degree 3 poles (247.9583, 3.1345) (247.9556, 3.0356) (247.9452, 2.9546) (247.9273, 2.8943) knots 0 0 0 0 1 1 1 1
  spline S432 degree 3 poles (247.9273, 2.8943) (247.909, 2.8323) (247.8868, 2.8058) (247.8716, 2.7959) knots 0 0 0 0 1 1 1 1
  spline S433 degree 3 poles (247.8716, 2.7959) (247.8613, 2.7895) (247.8392, 2.7809) (247.7873, 2.8013) knots 0 0 0 0 1 1 1 1
  spline S434 degree 3 poles (247.7873, 2.8013) (247.7333, 2.8226) (247.6587, 2.8718) (247.561, 2.9635) knots 0 0 0 0 1 1 1 1
  spline S435 degree 3 poles (242.2739, 16.5932) (241.8716, 16.9277) (241.4634, 16.9441) (241.1212, 16.8238) knots 0 0 0 0 1 1 1 1
  spline S436 degree 3 poles (241.1212, 16.8238) (240.8899, 16.7425) (240.6905, 16.5999) (240.5409, 16.4563) knots 0 0 0 0 1 1 1 1
  line L55 (240.5409, 16.4563) -> (240.5409, 17.472)
  spline S437 degree 3 poles (240.5409, 17.472) (240.6548, 17.44) (240.782, 17.4278) (240.9137, 17.4288) knots 0 0 0 0 1 1 1 1
  spline S438 degree 3 poles (240.9137, 17.4288) (241.1024, 17.4302) (241.3078, 17.4585) (241.51, 17.5008) knots 0 0 0 0 1 1 1 1
  spline S439 degree 3 poles (241.51, 17.5008) (241.8632, 17.5747) (242.2141, 17.6927) (242.462, 17.7918) knots 0 0 0 0 1 1 1 1
  spline S440 degree 3 poles (242.462, 17.7918) (242.5554, 17.4435) (242.6415, 17.0095) (242.6326, 16.7175) knots 0 0 0 0 1 1 1 1
  spline S441 degree 3 poles (242.6326, 16.7175) (242.6301, 16.638) (242.6206, 16.5744) (242.6052, 16.5283) knots 0 0 0 0 1 1 1 1
  spline S442 degree 3 poles (242.6052, 16.5283) (242.5896, 16.4815) (242.5717, 16.4636) (242.5601, 16.457) knots 0 0 0 0 1 1 1 1
  spline S443 degree 3 poles (242.5601, 16.457) (242.551, 16.4519) (242.5295, 16.4447) (242.4812, 16.4615) knots 0 0 0 0 1 1 1 1
  spline S444 degree 3 poles (242.4812, 16.4615) (242.4315, 16.4789) (242.3633, 16.5188) (242.2739, 16.5932) knots 0 0 0 0 1 1 1 1
  spline S445 degree 3 poles (251.3167, 2.3472) (251.5746, 2.6685) (251.9575, 3.1054) (252.2521, 3.4328) knots 0 0 0 0 1 1 1 1
  spline S446 degree 3 poles (252.2521, 3.4328) (252.5433, 3.2317) (253.0093, 3.0236) (253.571, 2.877) knots 0 0 0 0 1 1 1 1
  spline S447 degree 3 poles (253.571, 2.877) (254.1828, 2.7174) (254.9154, 2.6287) (255.6721, 2.7043) knots 0 0 0 0 1 1 1 1
  spline S448 degree 3 poles (255.6721, 2.7043) (255.7872, 2.7159) (255.8771, 2.7168) (255.9456, 2.7103) knots 0 0 0 0 1 1 1 1
  spline S449 degree 3 poles (255.9456, 2.7103) (256.0151, 2.7035) (256.0561, 2.6894) (256.0786, 2.6759) knots 0 0 0 0 1 1 1 1
  spline S450 degree 3 poles (256.0786, 2.6759) (256.0978, 2.6643) (256.101, 2.655) (256.1024, 2.648) knots 0 0 0 0 1 1 1 1
  spline S451 degree 3 poles (256.1024, 2.648) (256.1044, 2.6365) (256.1033, 2.6137) (256.0866, 2.5755) knots 0 0 0 0 1 1 1 1
  spline S452 degree 3 poles (256.0866, 2.5755) (256.0527, 2.4981) (255.9719, 2.3957) (255.8507, 2.2789) knots 0 0 0 0 1 1 1 1
  spline S453 degree 3 poles (255.8507, 2.2789) (255.7394, 2.1719) (255.6008, 2.0585) (255.4496, 1.9486) knots 0 0 0 0 1 1 1 1
  spline S454 degree 3 poles (255.4496, 1.9486) (254.8283, 2.0589) (253.8866, 2.1975) (253.0284, 2.2637) knots 0 0 0 0 1 1 1 1
  spline S455 degree 3 poles (253.0284, 2.2637) (252.5903, 2.2976) (252.1715, 2.3128) (251.827, 2.2951) knots 0 0 0 0 1 1 1 1
  spline S456 degree 3 poles (251.827, 2.2951) (251.6549, 2.2864) (251.4993, 2.2692) (251.368, 2.2413) knots 0 0 0 0 1 1 1 1
  spline S457 degree 3 poles (251.368, 2.2413) (251.3068, 2.2284) (251.2491, 2.2128) (251.1966, 2.1935) knots 0 0 0 0 1 1 1 1
  spline S458 degree 3 poles (251.1966, 2.1935) (251.2314, 2.2396) (251.2718, 2.2911) (251.3167, 2.3472) knots 0 0 0 0 1 1 1 1
extrude "Extrude3" add sketch "Sketch3" along normal blind 1.6 separate body contours S0 S1 S2 S3 S4 S5 S6 S7 S8 S9 S10 S11 S12 L0 S13 S14 S15 S16 S17 L1 S18 S19 S20 S21 S22 S23 S24 S25 S26 S27 S33 S34 S404 L52 S405 S406 | S25 L2 S26 S33 S34 | S25 L2 S26 S28 S29 S30 S31 S32 S33 S34 S35 S36 S37 L3 | S10 L5 S403 S404 S406 S407 | S10 S404 L52 S405 S406 | L5 S403 S407 S408 S409 S410 S411 S412 | S50 S51 S52 S53 S54 S55 S56 S57 S58 S61 S62 S63 S64 S65 L5 S71 S72 L10 S403 S407 S408 S409 S410 S411 S412 | S58 S59 S60 S61 S71 S72 L10 | S58 S59 S60 S61 S66 L6 L8 L9 S67 S68 S69 S70 S71 L10 L11 L12 S73 S74 L13 L14 S75 S76 S89 S90 | L6 L7 L8 L21 S89 S90 L22 | L7 S82 L15 L16 L17 L18 S83 S84 S85 S86 S87 S88 L19 L20 L21 L22 L23 S91 S92 S436 L55 S437 S438 | S83 S84 S436 L55 S437 S438 | S83 S84 S113 S435 S436 S438 S439 | S98 S99 S100 S101 S102 S103 S104 S105 S106 S107 S108 S109 S110 S111 S112 S113 S114 S115 S116 S117 S118 S119 L24 S435 S439 S440 S441 S442 S443 S444 | S113 S435 S439 S440 S441 S442 S443 S444 | S42 S43 S44 S45 S46 S47 S48 S49 | S120 S121 S122 S123 S124 S126 S127 S128 S129 S130 S131 S132 S133 S134 S135 S136 S137 L25 S138 S139 S140 L26 S141 S142 S143 S144 S160 | S124 S125 S126 S145 S146 S147 S148 S149 S150 S151 S152 S153 S154 S156 S157 S158 S159 S160 S161 S162 S163 S164 S165 S166 L27 S189 S190 L28 | S124 S125 S126 S160 | S154 S155 S156 S189 S190 L28 | S154 S155 S156 S175 S176 S177 S178 S179 S180 S181 S182 S183 S187 S188 S189 L28 L31 | S183 S184 S185 S186 S187 L31 | S183 S184 S185 S186 S187 L29 S191 S192 S193 S194 S195 L30 L31 S196 S197 S198 S199 S200 S201 S202 S203 S204 S206 S207 S208 S224 | S204 S205 S206 S224 | S204 S205 S206 S209 S210 S211 S212 S213 S214 S215 S216 S217 S218 S219 S220 S221 S222 S223 S224 S225 S226 S227 S228 S229 S230 L32 | S167 S168 S169 S170 S171 S172 S173 S174 | L33 S231 S232 S233 S234 S235 S236 S237 S238 S239 S240 S241 S242 S243 S244 S245 S246 S247 S248 L34 S249 S250 S251 S252 S253 S254 S255 S256 S257 S258 S259 S260 S261 S262 S263 S264 L35 S265 S266 S415 L53 S416 S417 | S241 S287 S288 S413 S414 S415 S417 S418 | S241 S415 L53 S416 S417 | S287 S288 S413 S418 S419 S420 S421 S422 S423 | S272 S273 S274 S275 S276 S277 S278 S279 S280 S281 S283 S284 S285 S286 S287 S288 S289 S290 S291 S292 S293 L37 S300 S301 L38 S413 S418 S419 S420 S421 S422 S423 | S281 S282 S283 S300 S301 L38 | S281 S282 S283 S294 S295 S296 S297 S298 S299 S300 L38 S302 S303 L39 S304 S305 S306 S307 S308 S309 S310 S426 L54 S427 | S296 S297 S426 L54 S427 | S296 S297 S322 S323 S424 S425 S426 S427 S428 S429 | S315 S316 S317 S318 S319 S320 S321 S322 S323 S324 S325 S326 L40 S327 S424 S429 S430 S431 S432 S433 S434 S445 S446 S455 S456 S457 S458 | S322 S323 S424 S429 S430 S431 S432 S433 S434 | S318 S319 S445 S446 S455 S456 S457 S458 | S318 S319 S346 S446 S447 S454 S455 | S336 S337 S338 S339 S342 S343 S344 S345 S346 S347 S348 S349 S350 S351 S352 L42 S353 S354 S355 S356 L43 S357 S358 S359 L46 S447 S448 S449 S450 S451 S452 S453 S454 | S346 S447 S448 S449 S450 S451 S452 S453 S454 | S339 S340 S341 S342 L46 | S339 S340 S341 S342 L44 S360 S361 S362 S363 S364 L45 L46 S365 S366 S367 S368 S369 S370 S371 S372 S373 S375 S376 S377 S389 | S373 S374 S375 S389 | S373 S374 S375 S378 S379 S380 L47 S381 L48 S382 L49 S383 S384 S385 S386 S387 S388 S389 S390 S391 | S267 S268 S269 L36 S270 S271 makes body 16 at (238.1249, 18.7957, 0) makes body 17 at (229.9079, 7.2036, 0) makes body 18 at (251.6833, 19.7721, 0) makes body 19 at (231.0078, 24.0195, 0) makes body 20 at (265.1789, 24.0195, 0)